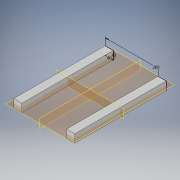
# Autodesk Inventor part: Assembly Mount Rack
Saved by Autodesk Inventor 2019 (Build 230136000, 136)
## iProperties
Created: 2021-02-18
Part Number: Assembly Mount Rack
Material: Generic
Document SubType Name: Modeling
Designer: Eric
Density: 1 g/cm^3
Appearance: Default
Author: Eric
Autodesk Inventor part; units mm, degrees
ref_plane "YZ Plane" through (0, 0, 0) normal (1, 0, 0) x (0, 1, 0)
ref_plane "XZ Plane" through (0, 0, 0) normal (0, 1, 0) x (-1, 0, 0)
ref_plane "XY Plane" through (0, 0, 0) normal (0, 0, 1) x (1, 0, 0)
sketch "Sketch1" plane through (0, 0, 0) normal (0, 0, 1) x (1, 0, 0)
  line L0 (0, 0) -> (40, 0)
  line L1 (40, 0) -> (40, -40)
  line L2 (40, -40) -> (0, -40)
  line L3 (0, -40) -> (0, 0)
  line L4 (260, 0) -> (300, 0)
  line L5 (300, 0) -> (300, -40)
  line L6 (300, -40) -> (260, -40)
  line L7 (260, -40) -> (260, 0)
  dimension "d0" = 40
  dimension "d1" = 40
  dimension "d2" = 260
  constraints: 16 end point, 4 horizontal, 4 vertical, 2 equal length, 1 collinear
  measures "d0" distance of L1.end L2.end
  measures "d1" distance of L0.end L1.end
  measures "d2" distance of L4.start L0.start
extrude "Extrusion1" add sketch "Sketch1" along normal blind 450 contours L0 L1 L2 L3
extrude "Extrusion2" add sketch "Sketch1" along normal up to surface (450 mm away) separate body contours L4 L5 L6 L7
ref_plane "Work Plane1" through (0, 0, 225) normal (0, 0, 1) x (1, 0, 0)
ref_plane "Work Plane2" through (150, -40, 0) normal (1, 0, 0) x (0, 0, -1)
ref_plane "Work Plane3" through (0, -20, 0) normal (0, 1, 0) x (1, 0, 0)
body "Solid1"
body "Solid2"
